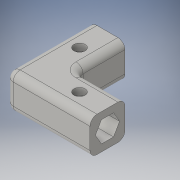
# Autodesk Inventor part: 3_8_angleJoint
Saved by Autodesk Inventor 2016 SP1 (Build 200210100, 210)
## iProperties
Created: 2015-11-23
Part Number: 3_8_angleJoint
Material: Generic
Document SubType Name: Modeling
Designer: steele
Density: 1 g/cm^3
Appearance: Default
Author: steele
Autodesk Inventor part; units mm, degrees
ref_plane "YZ Plane" through (0, 0, 0) normal (1, 0, 0) x (0, 1, 0)
ref_plane "XZ Plane" through (0, 0, 0) normal (0, 1, 0) x (-1, 0, 0)
ref_plane "XY Plane" through (0, 0, 0) normal (0, 0, 1) x (1, 0, 0)
sketch "Sketch1" plane through (0, 0, 0) normal (0, 1, 0) x (-1, 0, 0)
  line L0 (0, 0) -> (0, -22.225)
  line L1 (0, -22.225) -> (15.875, -22.225)
  line L2 (15.875, -22.225) -> (15.875, 15.875)
  line L3 (15.875, 15.875) -> (-22.225, 15.875)
  line L4 (-22.225, 15.875) -> (-22.225, 0)
  line L5 (-22.225, 0) -> (0, 0)
  dimension "d0" = 15.875
  dimension "d1" = 38.1
  constraints: 12 end point, 7 perpendicular, 1 vertical
  measures "d0" distance of L0.end L1.end
  measures "d1" distance of L1.end L2.end
extrude "Extrusion1" add sketch "Sketch1" against normal blind 15.875
sketch "Sketch3" plane through (0, 0, -22.225) normal (0, 0, -1) x (-1, 0, 0)
  line L0 (5.1879, -3.175) -> (10.6871, -3.175)
  line L1 (10.6871, -3.175) -> (13.4368, -7.9375)
  line L2 (13.4368, -7.9375) -> (10.6871, -12.7)
  line L3 (10.6871, -12.7) -> (5.1879, -12.7)
  line L4 (5.1879, -12.7) -> (2.4382, -7.9375)
  line L5 (2.4382, -7.9375) -> (5.1879, -3.175)
  line L6 (15.875, -15.875) -> (0, -15.875) projected
  line L7 (0, 0) -> (0, -15.875) projected
  point P0 (7.9375, -7.9375)
  dimension "d5" = 7.9375
  dimension "d6" = 7.9375
  dimension "d7" = 9.525
  constraints: 12 end point, 1 parallel, 13 other
  measures "d5" distance from line of L7 point (7.938, -7.938)
  measures "d6" distance from line of point (7.938, -7.938) L6
  measures "d7" distance between parallel lines of L0 L3
extrude "Extrusion2" cut sketch "Sketch3" against normal blind 31.75
sketch "Sketch4" plane through (22.225, 0, 15.875) normal (1, 0, 0) x (0, 0, -1)
  line L0 (13.4368, -7.9375) -> (10.6871, -12.7)
  line L1 (10.6871, -12.7) -> (5.1879, -12.7)
  line L2 (5.1879, -12.7) -> (2.4382, -7.9375)
  line L3 (2.4382, -7.9375) -> (5.1879, -3.175)
  line L4 (5.1879, -3.175) -> (10.6871, -3.175)
  line L5 (10.6871, -3.175) -> (13.4368, -7.9375)
  line L6 (0, 0) -> (15.875, 0) projected
  line L7 (15.875, 0) -> (15.875, -15.875) projected
  point P0 (7.9375, -7.9375)
  dimension "d10" = 9.525
  dimension "d11" = 7.9375
  dimension "d12" = 7.9375
  constraints: 12 end point, 1 parallel, 13 other
  measures "d10" distance between parallel lines of L1 L4
  measures "d11" distance from line of L7 point (7.938, -7.938)
  measures "d12" distance from line of point (7.938, -7.938) L6
extrude "Extrusion3" cut sketch "Sketch4" against normal blind 31.75
sketch "Sketch5" plane through (0, 0, 0) normal (0, 1, 0) x (1, 0, 0)
  line L0 (-15.875, 22.225) -> (-15.875, -15.875) projected
  line L1 (-15.875, -15.875) -> (22.225, -15.875) projected
  line L2 (0, 22.225) -> (-15.875, 22.225) projected
  line L3 (22.225, -15.875) -> (22.225, 0) projected
  point P0 (0, 0)
  point P1 (-7.9375, 9.525)
  point P2 (9.525, -7.9375)
  dimension "d15" = 7.9375
  dimension "d16" = 7.9375
  dimension "d17" = 12.7
  dimension "d18" = 12.7
  measures "d15" distance from line of point (-7.938, 9.525) L0
  measures "d16" distance from line of L1 point (9.525, -7.938)
  measures "d17" distance from line of point (-7.938, 9.525) L2
  measures "d18" distance from line of point (9.525, -7.938) L3
hole "Hole1" at (-7.9375, 0, -9.525) at (9.525, 0, 7.9375) direction (0, -1, 0) diameter 5.1054 end through all clearance for "Flat Head Machine Screw (82)" size "#10" standard "Ansi Unified Screw Threads"
fillet "Fillet1" radius 3.175 6 edges at (-15.875, -7.9375, 15.875) (0, -7.9375, 0) (11.1125, 0, 0) (0, 0, -11.1125) (3.175, 0, 15.875) (-15.875, 0, -3.175)
fillet "Fillet2" radius 3.175 6 edges at (-14.9451, -15.875, 14.9451) (4.7625, -15.875, 15.875) (-15.875, -15.875, -4.7625) (0.9299, -15.875, -0.9299) (12.7, -15.875, 0) (0, -15.875, -12.7)
equation "\"d0\" = pieceWidth"
equation "\"d1\" = pieceLength"
equation "\"d2\" = pieceWidth"
equation "\"d5\" = 0.5 * pieceWidth"
equation "\"d6\" = 0.5 * pieceWidth"
equation "\"d7\" = hex"
equation "\"d8\" = depthOfHexCut"
equation "\"d10\" = hex"
equation "\"d11\" = 0.5 * pieceWidth"
equation "\"d12\" = 0.5 * pieceWidth"
equation "\"d13\" = depthOfHexCut"
equation "\"d15\" = 0.5 * pieceWidth"
equation "\"d16\" = 0.5 * pieceWidth"
equation "\"d17\" = 0.5 * depthOfInsert"
equation "\"d18\" = 0.5 * depthOfInsert"
equation "\"hex\" = 9.525"
equation "\"pieceWidth\" = 15.875"
equation "\"pieceLength\" = 38.1"
equation "\"depthOfInsert\" = 25.4"
equation "\"depthOfHexCut\" = 31.75"
body "Solid1"
